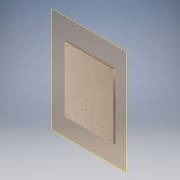
# Autodesk Inventor part: Metal_sheet
Saved by Autodesk Inventor 2019 (Build 230136000, 136)
## iProperties
Created: 2021-02-06
Part Number: Metal_sheet
Material: Aluminum 6061
Document SubType Name: Modeling
Designer: rtavi
Density: 2.7 g/cm^3
Appearance: Aluminum - Flat
Mass: 810 g
Surface Area: 3032 cm^2
Volume: 300 cm^3
Author: rtavi
Autodesk Inventor part; units mm, degrees
ref_plane "YZ Plane" through (0, 0, 0) normal (1, 0, 0) x (0, 1, 0)
ref_plane "XZ Plane" through (0, 0, 0) normal (0, 1, 0) x (-1, 0, 0)
ref_plane "XY Plane" through (0, 0, 0) normal (0, 0, 1) x (1, 0, 0)
ref_plane "Work Plane1" through (0, 0, 0) normal (0, 0, 1) x (1, 0, 0)
sketch "Sketch1" plane through (0, 0, 0) normal (0, 0, 1) x (1, 0, 0)
  line L0 (-150, -200) -> (150, -200)
  line L1 (150, -200) -> (150, 200)
  line L2 (150, 200) -> (-150, 200)
  line L3 (-150, 200) -> (-150, -200)
  line L4 (0, -280) -> (0, 280) construction
  line L5 (-210, 0) -> (210, 0) construction
  point P0 (0, 0)
  dimension "d0" = 400
  dimension "d1" = 300
  constraints: 8 end point, 2 parallel, 1 horizontal, 1 perpendicular, 2 other
  measures "d0" distance of L2.end L0.start
  measures "d1" distance between parallel lines of L1 L3
extrude "Extrusion1" add sketch "Sketch1" against normal blind 12
sketch "Sketch2" plane through (0, 0, -12) normal (0, 0, 1) x (1, 0, 0)
  line L0 (0, 0) -> (-281.1142, 0) construction
  line L1 (0, 0) -> (0, -490.5016) construction
  line L2 (-150, -200) -> (150, -200) construction
  line L3 (-106.6853, -185) -> (102.3994, -185) construction
  line L4 (-96.6591, -157) -> (112.4256, -157) construction
  circle A0 centre (-82.5, -144) radius 2.15 construction
  circle A1 centre (-107.5, -144) radius 2.15 construction
  circle A2 centre (-107.5, 144) radius 2.15 construction
  circle A3 centre (-82.5, 144) radius 2.15 construction
  circle A4 centre (82.5, 144) radius 2.15 construction
  circle A5 centre (107.5, 144) radius 2.15 construction
  circle A6 centre (82.5, -144) radius 2.15 construction
  circle A7 centre (107.5, -144) radius 2.15 construction
  point P0 (-22.5, -157)
  point P1 (-34, -185)
  point P2 (22.5, -157)
  point P3 (34, -185)
  point P4 (-22.5, 157)
  point P5 (-34, 185)
  point P6 (34, 185)
  point P7 (22.5, 157)
  dimension "d8" = 15
  dimension "d9" = 28
  dimension "d10" = 22.5
  dimension "d11" = 34
  constraints: 8 centre point, 8 coincident, 8 end point, 6 symmetric about line, 3 horizontal, 2 point on line, 1 parallel, 1 vertical, 16 other
  measures "d8" distance between parallel lines of L2 L3
  measures "d9" distance between parallel lines of L4 L3
  measures "d10" distance from line of L1 point (-22.5, -157)
  measures "d11" distance from line of L1 point (-34, -185)
hole "Hole2" at (-22.5, -157, -12) at (-34, -185, -12) at (34, -185, -12) at (22.5, -157, -12) at (-22.5, 157, -12) at (22.5, 157, -12) at (34, 185, -12) at (-34, 185, -12) at (107.5, -144, -12) at (82.5, -144, -12) at (-82.5, -144, -12) at (-107.5, -144, -12) at (-107.5, 144, -12) at (-82.5, 144, -12) at (82.5, 144, -12) at (107.5, 144, -12) direction (0, 0, 1) diameter 4.1 end through all counterbore diameter 7.2 counterbore depth 4.1
sketch "Sketch3" plane through (0, 0, -12) normal (0, 0, -1) x (-1, 0, 0)
  line L0 (-150, -200) -> (150, -200) construction
  line L1 (150, -200) -> (150, 200) construction
  line L2 (-150, 200) -> (-150, -200) construction
  line L3 (150, 200) -> (-150, 200) construction
  line L4 (135, -185) -> (-135, -185) construction
  line L5 (-135, -185) -> (-135, 185) construction
  line L6 (-135, 185) -> (135, 185) construction
  line L7 (135, 185) -> (135, -185) construction
  point P0 (0, 0)
  dimension "d29" = 15
  constraints: 8 end point, 4 coincident, 3 other
  measures "d29" distance between parallel lines of L0 L4
hole "Hole3" at (-135, -185, -12) at (-135, 185, -12) at (135, 185, -12) at (135, -185, -12) direction (0, 0, 1) diameter 8.2 end through all
sketch "Sketch6" plane through (0, 0, -12) normal (0, 0, 1) x (1, 0, 0)
  line L0 (-27.5, -40) -> (27.5, -40) construction
  arc A0 (30.5, -43) -> (27.5, -40) centre (27.5, -43) ccw construction
  line L1 (30.5, -43) -> (30.5, -107) construction
  arc A1 (27.5, -110) -> (30.5, -107) centre (27.5, -107) ccw construction
  line L2 (27.5, -110) -> (-27.5, -110) construction
  arc A2 (-30.5, -107) -> (-27.5, -110) centre (-27.5, -107) ccw construction
  line L3 (-30.5, -107) -> (-30.5, -43) construction
  arc A3 (-27.5, -40) -> (-30.5, -43) centre (-27.5, -43) ccw construction
  circle A4 centre (-20.5, -75) radius 3.1 construction
  circle A5 centre (20.5, -50) radius 3.1 construction
  circle A6 centre (-20.5, -100) radius 3.1 construction
  circle A7 centre (-20.5, -50) radius 3.1 construction
  circle A8 centre (20.5, -100) radius 3.1 construction
  circle A9 centre (20.5, -75) radius 3.1 construction
  constraints: 10 centre point, 8 end point, 8 point on circle, 2 horizontal, 2 vertical, 28 other
hole "Hole6" at (-20.5, -100, -12) at (20.5, -100, -12) at (20.5, -75, -12) at (20.5, -50, -12) at (-20.5, -75, -12) at (-20.5, -50, -12) direction (0, 0, 1) diameter 6.2 end through all counterbore diameter 10.2 counterbore depth 6.2
body "Solid1"
